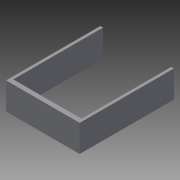
# Autodesk Inventor part: 知能ロボコン大砲５
Saved by Autodesk Inventor 2013 (Build 170138000, 138)
## iProperties
Created: 2014-05-12
Part Number: 知能ロボコン大砲５
Material: 一般
Document SubType Name: Modeling
Designer: horumo136
Density: 1 g/cm^3
Author: horumo136
Autodesk Inventor part; units mm, degrees
ref_plane "YZ Plane" through (0, 0, 0) normal (1, 0, 0) x (0, 1, 0)
ref_plane "XZ Plane" through (0, 0, 0) normal (0, 1, 0) x (-1, 0, 0)
ref_plane "XY Plane" through (0, 0, 0) normal (0, 0, 1) x (1, 0, 0)
sketch "スケッチ1" plane through (0, 0, 0) normal (0, 1, 0) x (-1, 0, 0)
  line L0 (-0.3902, 0.2385) -> (-82.3902, 0.2385)
  line L1 (-82.3902, 0.2385) -> (-82.3902, 30.2385)
  line L2 (-82.3902, 30.2385) -> (-0.3902, 30.2385)
  line L3 (-0.3902, 30.2385) -> (-0.3902, 0.2385)
  point P0 (0, 0)
  dimension "d0" = 82
  dimension "d1" = 30
  constraints: 8 end point, 2 parallel, 1 horizontal, 1 perpendicular
  measures "d0" distance of L1.end L2.end
  measures "d1" distance of L0.end L1.end
extrude "押し出し1" add sketch "スケッチ1" along normal blind 5
sketch "スケッチ2" plane through (0, 5, 0) normal (0, 1, 0) x (1, 0, 0)
  line L0 (82.3902, -0.2385) -> (0.3902, -0.2385) projected
  line L1 (0.3902, -30.2385) -> (82.3902, -30.2385) projected
  line L2 (0.3902, -0.2385) -> (3.3902, -0.2385)
  line L3 (3.3902, -0.2385) -> (3.3902, -30.2385)
  line L4 (3.3902, -30.2385) -> (0.3902, -30.2385)
  line L5 (0.3902, -30.2385) -> (0.3902, -0.2385)
  line L6 (82.3902, -30.2385) -> (79.3902, -30.2385)
  line L7 (79.3902, -30.2385) -> (79.3902, -0.2385)
  line L8 (79.3902, -0.2385) -> (82.3902, -0.2385)
  line L9 (82.3902, -0.2385) -> (82.3902, -30.2385)
  point P0 (0, 0)
  dimension "d4" = 3
  dimension "d5" = 3
  constraints: 16 end point, 4 parallel, 2 horizontal, 2 perpendicular, 2 point on line
  measures "d4" distance of L3.end L4.end
  measures "d5" distance of L7.end L8.end
extrude "押し出し2" add sketch "スケッチ2" along normal blind 100 contours L9 L1 L7 L0 | L3 L1 L5 L0
